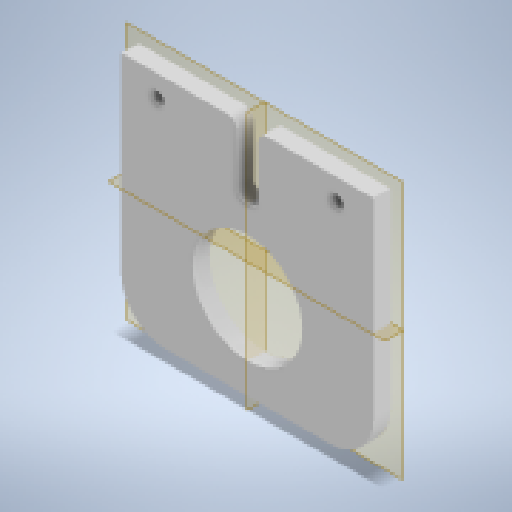
# Autodesk Inventor part: Скоба трубы
Saved by Autodesk Inventor 2023.2 (Build 272271030, 271C)
## iProperties
Created: 2024-04-14
Part Number: Скоба трубы
Material: Типовые
Document SubType Name: Modeling
Designer: I9232
Density: 1 g/cm^3
Appearance: По умолчанию
Author: I9232
Autodesk Inventor part; units mm, degrees
sketch "Эскиз1" plane through (0, 0, 0) normal (0, 0, 1) x (1, 0, 0)
  line L0 (-29.5, -27.5) -> (29.5, -27.5)
  line L1 (29.5, -27.5) -> (29.5, 27.5)
  line L2 (29.5, 27.5) -> (-29.5, 27.5)
  line L3 (-29.5, 27.5) -> (-29.5, -27.5)
  line L4 (-29.5, -27.5) -> (29.5, 27.5) construction
  line L5 (29.5, -27.5) -> (-29.5, 27.5) construction
  circle A0 centre (0, -7.5) radius 12.8
  line L6 (0, -7.5) -> (0, -27.5) construction
  circle A1 centre (-21.05, 22.5) radius 1.5
  circle A2 centre (21.05, 22.5) radius 1.5
  line L7 (-21.05, 22.5) -> (21.05, 22.5)
  point P0 (0, 0)
  dimension "d0" = 59
  dimension "d1" = 55
  dimension "d2" = 25.6
  dimension "d3" = 20
  dimension "d4" = 3
  dimension "d7" = 42.1
  dimension "d8" = 8.45
  dimension "d13" = 5
  constraints: 16 end point, 3 centre point, 3 midpoint, 2 horizontal, 2 parallel, 1 coincident, 1 equal radius, 1 perpendicular
  measures "d0" distance of L1.end L2.end
  measures "d1" distance of L0.end L1.end
  measures "d2" diameter of A0
  measures "d3" distance of L6.start L6.end
  measures "d4" diameter of A2
  measures "d7" distance of L7.start L7.end
  measures "d8" distance from line of L1 A2.centre
  measures "d13" distance from line of L2 A2.centre
extrude "Выдавливание1" add sketch "Эскиз1" along normal blind 4
sketch "Эскиз2" plane through (0, 0, 4) normal (0, 0, 1) x (1, 0, 0)
  line L0 (29.5, 27.5) -> (-29.5, 27.5) projected
  line L1 (-2.5247, 27.5) -> (-2.5247, 11.5)
  line L2 (2.5247, 27.5) -> (2.5247, 11.5)
  line L3 (-2.5247, 11.5) -> (2.5247, 11.5)
  point P0 (0, 0)
  dimension "d9" = 16
  constraints: 6 end point, 2 point on line, 1 horizontal, 1 vertical
  measures "d9" distance of L2.start L2.end
extrude "Выдавливание2" cut sketch "Эскиз2" against normal up to surface (4 mm away)
fillet "Сопряжение1" radius 2 4 edges at (2.5247, 11.5, 2) (-2.5247, 11.5, 2) (2.5247, 27.5, 2) (-2.5247, 27.5, 2)
sketch "Эскиз3" plane through (0, 0, 4) normal (0, 0, 1) x (1, 0, 0)
  line L0 (-29.5, 27.5) -> (-29.5, -27.5) projected
  line L1 (-29.5, -17.5) -> (-19.5, -17.5) construction
  line L2 (-19.5, -17.5) -> (-19.5, -27.5) construction
  line L3 (-29.5, -27.5) -> (29.5, -27.5) projected
  line L4 (-29.5, 27.5) -> (-29.5, -27.5) projected
  line L5 (-29.5, -27.5) -> (29.5, -27.5) projected
  line L6 (19.5, -27.5) -> (19.5, -17.5) construction
  line L7 (19.5, -17.5) -> (29.5, -17.5) construction
  line L8 (29.5, -27.5) -> (29.5, 27.5) projected
  arc A0 (-29.5, -17.5) -> (-19.5, -27.5) centre (-19.5, -17.5) ccw
  arc A1 (19.5, -27.5) -> (29.5, -17.5) centre (19.5, -17.5) ccw
  point P0 (0, 0)
  constraints: 8 end point, 4 perpendicular, 4 point on circle, 4 point on line, 2 centre point, 2 coincident, 1 horizontal, 1 vertical
extrude "Выдавливание3" cut sketch "Эскиз3" against normal up to surface (4 mm away)
